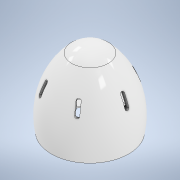
# Autodesk Inventor part: SmartEgg Shell Top
Saved by Autodesk Inventor 2020 (Build 240168000, 168)
## iProperties
Created: 2019-11-26
Part Number: SmartEgg Shell Top
Material: Generic
Document SubType Name: Modeling
Designer: Andrew
Density: 1 g/cm^3
Appearance: White
Author: Andrew
Autodesk Inventor part; units mm, degrees
ref_plane "YZ Plane" through (0, 0, 0) normal (1, 0, 0) x (0, 1, 0)
ref_plane "XZ Plane" through (0, 0, 0) normal (0, 1, 0) x (-1, 0, 0)
ref_plane "XY Plane" through (0, 0, 0) normal (0, 0, 1) x (1, 0, 0)
derived "SmartEgg Shell.ipt"
sketch "Shell Sketch" plane through (0, -10.304121, -14.021904) normal (0, 0.7989679, -0.6013737) x (0, 0.6013737, 0.7989679)
  arc A0 (41.04699, -18.667104) -> (29.65452, 33.515802) centre (-5.946947, -1.591684) ccw
  arc A1 (17.550021, -35.129394) -> (30.050021, -31.780029) centre (17.550021, -10.129394) ccw construction
  line L0 (17.550021, -35.129394) -> (17.550021, -31.780029) construction
  line L1 (17.550021, 9.75) -> (37.100043, 9.75)
  line L2 (17.550021, 26.5) -> (17.550021, -26.5) construction
  line L3 (35.100043, -26.5) -> (35.831294, -27.182109) construction
  arc A2 (29.65452, 33.515802) -> (17.550021, 38.579257) centre (17.550021, 21.579257) ccw
  line L4 (17.550021, 38.579257) -> (17.550021, 35.721392)
  line L5 (17.550021, 35.721392) -> (22.550021, 35.721392)
  arc A3 (28.230462, 32.111502) -> (22.550021, 35.721392) centre (17.550021, 21.579257) ccw
  arc A4 (39.288437, 14.463223) -> (28.230462, 32.111502) centre (-5.946947, -1.591684) ccw
  arc A5 (35.100043, 22) -> (30.600043, 26.5) centre (30.600043, 22) ccw construction
  line L6 (37.100043, 9.75) -> (37.100043, -11.780029)
  line L7 (37.100043, -11.780029) -> (43.004025, -11.780029)
  line L8 (40.100043, 9.75) -> (40.100043, -11.530029)
  line L9 (40.100043, -11.530029) -> (43.055393, -11.530029)
  line L10 (17.550021, -31.780029) -> (30.050021, -31.780029)
  arc A6 (30.050021, -31.780029) -> (41.04699, -18.667104) centre (17.550021, -10.129394) ccw
  line L11 (17.550021, -31.780029) -> (17.550021, 9.75)
  line L12 (35.100043, -26.5) -> (35.100043, 22) construction
  line L13 (20.707233, 10.75) -> (17.399678, 10.75) construction
  arc A7 (40.100043, 9.75) -> (39.288437, 14.463223) centre (26.008732, 9.75) ccw
  point P0 (17.399678, 0)
  point P1 (40.100043, 11.960982)
sketch "Thread Sketch" plane through (0, -10.304121, -14.021904) normal (0, 0.7989679, -0.6013737) x (0, 0.6013737, 0.7989679)
  line L0 (37.100043, 9.75) -> (37.100043, -11.780029) construction
  line L1 (40.100043, 9.75) -> (40.100043, -11.530029) construction
  line L2 (37.100043, 9.75) -> (39.600043, 7.25)
  line L3 (39.600043, 7.25) -> (39.600043, 5.25)
  line L4 (39.600043, 5.25) -> (37.100043, 2.75)
  line L5 (37.100043, 2.75) -> (37.100043, 9.75)
  line L6 (40.100043, 5.396447) -> (37.600043, 2.896447)
  line L7 (37.600043, 2.896447) -> (37.600043, 0.896447)
  line L8 (37.600043, 0.896447) -> (40.100043, -1.603553)
  line L9 (40.100043, -1.603553) -> (40.100043, 5.396447)
  line L10 (39.600043, 6.25) -> (37.100043, 6.25) construction
  line L11 (37.600043, 1.896447) -> (40.100043, 1.896447) construction
  point P0 (17.399678, 0)
sketch "Thread Mask" plane through (0, -10.304121, -14.021904) normal (0, 0.7989679, -0.6013737) x (0, 0.6013737, 0.7989679)
  line L0 (40.100043, 7.25) -> (37.100043, 7.25)
  line L1 (37.100043, 7.25) -> (37.100043, -11.780029)
  line L2 (37.100043, -11.780029) -> (40.100043, -11.780029)
  line L3 (40.100043, -11.780029) -> (40.100043, 7.25)
  line L4 (37.100043, 9.75) -> (37.100043, -11.780029) construction
  line L5 (40.100043, 9.75) -> (40.100043, -11.530029) construction
  point P0 (17.399678, 0)
ref_plane "Vent Plane" through (17.25, 13.971591, 18.230113) normal (-0.3768337, -0.557041, -0.7400687) x (0.8282752, -0.5603214, 0)
sketch "Vent Lookup" plane through (0, -10.304121, -14.021904) normal (0, 0.7989679, -0.6013737) x (0, 0.6013737, 0.7989679)
  arc A0 (41.04699, -18.667104) -> (29.65452, 33.515802) centre (-5.946947, -1.591684) ccw
  line L0 (40.3671, 17.25) -> (17.550021, 7.967456)
  line L1 (17.550021, 26.5) -> (17.550021, -26.5) construction
  line L2 (20.707233, 10.75) -> (17.399678, 10.75) construction
  point P0 (17.399678, 0)
revolve "Revolution1" add sketch "Shell Sketch" angle 360 about axis through (-31.780029, 0.25, 0) along (1, 0, 0) contours L9 L8 A7 A4 A3 L5 L4 A2 A0
coil "Coil1" sketch "Thread Sketch" operation add axis through (-31.780029, 0.25, 0) along (-1, 0, 0) pitch 8.708 turns 3 hand right separate body contours L9 L8 L7 L6
coil "Coil2" sketch "Thread Sketch" operation add axis through (-31.780029, 0.25, 0) along (1, 0, 0) pitch 8.708 turns 3 hand right bodies 2 contours L9 L8 L7 L6
sketch "Top Thread Mask" plane through (0, -10.304121, -14.021904) normal (0, 0.7989679, -0.6013737) x (0, 0.6013737, 0.7989679)
  arc A0 (40.100043, 9.75) -> (39.288437, 14.463223) centre (26.008732, 9.75) ccw
  arc A1 (39.288437, 14.463223) -> (28.230462, 32.111502) centre (-5.946947, -1.591684) ccw
  arc A2 (28.230462, 32.111502) -> (22.550021, 35.721392) centre (17.550021, 21.579257) ccw
  line L0 (17.550021, 35.721392) -> (22.550021, 35.721392)
  line L1 (17.550021, 35.721392) -> (17.550021, -11.530029)
  line L2 (17.550021, -11.530029) -> (40.100043, -11.530029)
  line L3 (40.100043, -11.530029) -> (40.100043, 9.75)
  line L4 (40.100043, -11.530029) -> (43.055393, -11.530029) construction
  point P0 (17.399678, 0)
  constraints: 6 end point, 2 vertical, 1 collinear, 1 perpendicular
revolve "Revolution2" cut sketch "Top Thread Mask" angle 360 about axis through (35.721392, 0.25, 0) along (-1, 0, 0) keep common part bodies 2
combine bodies "Combine1" operation type add bodies to combine 1 2
sketch "Sketch6" plane through (17.25, 13.971591, 18.230113) normal (-0.3768337, -0.557041, -0.7400687) x (0.8282752, -0.5603214, 0)
  line L0 (-3.353229, 1.678796) -> (3.353229, -1.678796) construction
  line L1 (-3.912828, 0.561053) -> (2.793631, -2.796539)
  line L2 (3.912828, -0.561053) -> (-2.793631, 2.796539)
  arc A0 (-2.793631, 2.796539) -> (-3.912828, 0.561053) centre (-3.353229, 1.678796) ccw
  arc A1 (2.793631, -2.796539) -> (3.912828, -0.561053) centre (3.353229, -1.678796) ccw
  line L3 (-32.921858, 16.482343) -> (1.476437, -0.739179)
  point P0 (-6.459166, 3.457161)
  point P1 (0, 0)
  point P2 (0, 0)
  point P3 (0, 0)
  point P4 (0, 0)
  dimension "d19" = 2.5
  dimension "d20" = 7.5
  constraints: 8 end point, 4 point on circle, 4 tangent, 2 centre point, 1 coincident, 1 collinear, 1 midpoint, 1 parallel
  measures "d19" distance between parallel lines of L2 L1
  measures "d20" distance of L0.start L0.end
extrude "Extrusion1" add sketch "Sketch6" along normal blind 10 separate body
pattern_circular "Circular Pattern1" count 6 over 360 about axis through (-1.591684, 0.25, 0) along (-1, 0, 0) bodies 3
combine bodies "Combine2" operation type subtract main body 1 bodies to subtract 3
ref_plane "Work Plane2" through (0, -10.304121, -14.021904) normal (0, 0.7989679, -0.6013737) x (0, 0.6013737, 0.7989679)
equation "\"d2\" = 2 * Thread_Pitch"
equation "\"d10\" = 2 * Thread_Pitch"
equation "\"Thread_Pitch\" = 4.354"
body "Solid1"
